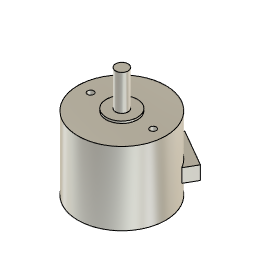
组装01-NIDEC+61mm飞轮 v2 (Autodesk Fusion 360 archive; units mm, degrees)
design "NIDEC无刷电机"
Autodesk Fusion 360 part; units mm, degrees
sketch "草图1" plane through (0, 0, 0) normal (0, 0, 1) x (1, 0, 0)
  circle A0 centre (0, 0) radius 21
  dimension "d1" = 42
  constraint coincident A0.centre origin
  measures "d1" diameter of A0
extrude "拉伸1" add sketch "草图1" along normal blind 35
sketch "草图2" plane through (0, 0, 35) normal (0, 0, 1) x (-1, 0, 0)
  circle A0 centre (0, 0) radius 21
  circle A1 centre (0, 0) radius 3
  dimension "d4" = 6
  constraint coincident A0.centre A1.centre
  measures "d4" diameter of A1
extrude "拉伸2" add sketch "草图2" along normal blind 18 contours A1
sketch "草图3" plane through (0, 0, 35) normal (0, 0, 1) x (-1, 0, 0)
  circle A0 centre (0, 0) radius 3
  circle A1 centre (0, 0) radius 21
  circle A2 centre (0, 0) radius 7.5
  dimension "d7" = 15
  constraint concentric A0 A2
  measures "d7" diameter of A2
extrude "拉伸3" add sketch "草图3" along normal blind 1 contours A2
sketch "草图4" plane through (0, 0, 35) normal (0, 0, 1) x (-1, 0, 0)
  circle A0 centre (0, 0) radius 7.5
  circle A1 centre (0, 0) radius 21
  circle A2 centre (0, 0) radius 15 construction
  circle A3 centre (15, -0.038) radius 1.5
  circle A4 centre (-15, 0) radius 1.5
  dimension "d10" = 30
  dimension "d11" = 3
  dimension "d12" = 3
  constraint coincident A0.centre A1.centre
  constraint coincident A2 A3.centre
  constraint coincident A2 A4.centre
  measures "d10" diameter of A2
  measures "d11" diameter of A3
  measures "d12" diameter of A4
extrude "拉伸4" cut sketch "草图4" against normal blind 10 contours A3 | A4
sketch "草图5" plane through (0, 0, 35) normal (0, 0, 1) x (-1, 0, 0)
  circle A0 centre (-15, 0) radius 1.5
  circle A1 centre (15, -0.038) radius 1.5
  circle A2 centre (0, 0) radius 7.5
  circle A3 centre (0, 0) radius 21
  line L0 (0, 0) -> (-15, 0) construction
  line L1 (-10.4937, -18.1902) -> (0, 0) construction
  line L2 (-0.5625, -20.9925) -> (-3.4002, -26.8403)
  line L3 (-3.4002, -26.8403) -> (-21.1573, -16.5965)
  line L4 (-21.1573, -16.5965) -> (-17.9093, -10.9662)
  dimension "d16" = 60.02
  dimension "d17" = 6.5
  dimension "d18" = 20.5
  constraint coincident A2.centre A3.centre
  constraint coincident A0.centre L0.end
  constraint coincident A3 L1.start
  constraint coincident A3 L2.start
  constraint coincident A3 L4.end
  constraint equal L2 L4
  constraint parallel L1 L4
  constraint perpendicular L1 L3
  measures "d16" angle of L0 L1
  measures "d17" distance of L2.start L2.end
  measures "d18" distance of L2.end L3.end
ref_plane "工作平面2" through (0, 0, 15) normal (0, 0, -1) x (-1, 0, 0)
sketch "草图6" plane through (0, 0, 15) normal (0, 0, -1) x (1, 0, 0)
  line L0 (10.2887, -17.835) -> (0, 0)
  line L1 (0, 0) -> (15, 0)
  line L2 (0.2802, -20.9981) -> (3.5282, -26.6284)
  line L3 (3.5282, -26.6284) -> (21.2853, -16.3846)
  line L4 (18.0373, -10.7543) -> (21.2853, -16.3846)
  circle A0 centre (0, 0) radius 21
  dimension "d23" = 60.02
  dimension "d24" = 6.5
  dimension "d25" = 6.5
  dimension "d26" = 20.5
  constraint coincident L0.end L1.start
  constraint horizontal L1
  constraint parallel L2 L4
  constraint parallel L0 L2
  constraint perpendicular L0 L3
  constraint coincident L2.start A0
  constraint coincident L4.start A0
  measures "d23" angle of L0 L1
  measures "d24" distance of L2.start L2.end
  measures "d25" distance of L3.end L4.start
  measures "d26" distance of L2.end L3.end
extrude "拉伸6" add sketch "草图6" along normal blind 6.5 contours L2 L3 L4 A0

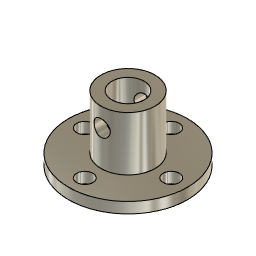
design "联轴器-6mm孔径"
Autodesk Fusion 360 part; units mm, degrees
sketch "草图1" plane through (0, 0, 0) normal (0, 0, 1) x (1, 0, 0)
  circle A0 centre (0, 0) radius 11
  dimension "d1" = 22
  constraint coincident A0.centre origin
  measures "d1" diameter of A0
extrude "拉伸1" add sketch "草图1" along normal blind 2
sketch "草图2" plane through (0, 0, 2) normal (0, 0, 1) x (-1, 0, 0)
  circle A0 centre (0, 0) radius 11
  circle A1 centre (0, 0) radius 5
  constraint concentric A0 A1
extrude "拉伸2" add sketch "草图2" along normal blind 10 contours A1
sketch "草图3" plane through (0, 0, 12) normal (0, 0, 1) x (-1, 0, 0)
  circle A0 centre (0, 0) radius 5
  circle A1 centre (0, 0) radius 3
  dimension "d6" = 6
  constraint concentric A0 A1
  measures "d6" diameter of A1
extrude "拉伸3" cut sketch "草图3" against normal blind 12 contours A1
sketch "草图4" plane through (0, 0, 2) normal (0, 0, 1) x (-1, 0, 0)
  circle A0 centre (0, 0) radius 5
  circle A1 centre (0, 0) radius 11
  circle A2 centre (0, 0) radius 8 construction
  circle A3 centre (8, 0.0048) radius 1.5
  circle A4 centre (-0.0048, 8) radius 1.5
  circle A5 centre (-8, -0.0048) radius 1.5
  circle A6 centre (0.0048, -8) radius 1.5
  dimension "d9" = 16
  dimension "d10" = 3
  dimension "d12" = 360
  constraint coincident A0.centre A1.centre
  constraint coincident A2 A3.centre
  measures "d9" diameter of A2
  measures "d10" diameter of A3
extrude "拉伸4" cut sketch "草图4" against normal blind 2 contours A3 | A4 | A5 | A6
sketch "草图5" plane through (0, 0, 0) normal (0, 1, 0) x (1, 0, 0)
  circle A0 centre (0, -8.5) radius 1.5
  dimension "d15" = 3
  measures "d15" diameter of A0
extrude "拉伸5" cut sketch "草图5" along normal mid plane 11

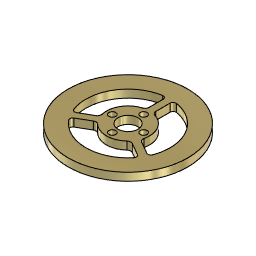
design "惯性飞轮-61mm直径"
Autodesk Fusion 360 part; units mm, degrees
sketch "草图1" plane through (0, 0, 0) normal (0, 0, 1) x (1, 0, 0)
  circle A0 centre (0, 0) radius 30.5
  circle A1 centre (-8, 0) radius 1.75
  line L0 (0, 0) -> (-11, 0)
  circle A2 centre (0, 0) radius 5.1
  circle A3 centre (0, -8) radius 1.75
  circle A4 centre (8, 0) radius 1.75
  circle A5 centre (0, 8) radius 1.75
  line L1 (-1.75, 21.4287) -> (-1.75, 10.8599)
  line L2 (1.75, 21.4287) -> (1.75, 10.8599)
  line L3 (-17.6828, -12.2299) -> (-8.53, -6.9455)
  line L4 (19.4328, -9.1988) -> (10.28, -3.9144)
  line L5 (-19.4328, -9.1988) -> (-10.28, -3.9144)
  line L6 (17.6828, -12.2299) -> (8.53, -6.9455)
  arc A6 (19.4328, -9.1988) -> (1.75, 21.4287) centre (0, 0) ccw
  arc A7 (-1.75, 21.4287) -> (-19.4328, -9.1988) centre (0, 0) ccw
  arc A8 (-17.6828, -12.2299) -> (17.6828, -12.2299) centre (0, 0) ccw
  arc A9 (-8.53, -6.9455) -> (8.53, -6.9455) centre (0, 0) ccw
  arc A10 (10.28, -3.9144) -> (1.75, 10.8599) centre (0, 0) ccw
  arc A11 (-1.75, 10.8599) -> (-10.28, -3.9144) centre (0, 0) ccw
  dimension "d1" = 61
  dimension "d2" = 43
  dimension "d3" = 22
  dimension "d4" = 3.5
  dimension "d5" = 10.2
  dimension "d6" = 8
  dimension "d8" = 360
  dimension "d9" = 3.5
  dimension "d12" = 360
  dimension "d14" = 360
  constraint coincident A0.centre L0.start
  constraint concentric A7 A9
  constraint coincident L0.end A9
  constraint horizontal L0
  constraint coincident A1.centre L0
  constraint concentric A2 A9
  constraint coincident L1.end A9
  constraint vertical L1
  constraint coincident L2.end A9
  constraint parallel L1 L2
  constraint concentric A6 A7
  constraint concentric A7 A8
  constraint concentric A9 A10
  constraint concentric A10 A11
  measures "d1" diameter of A0
  measures "d2" diameter of A7
  measures "d3" diameter of A9
  measures "d4" diameter of A1
  measures "d5" diameter of A2
  measures "d6" distance of A1.centre A0.centre
  measures "d9" distance of L1 L2
extrude "拉伸1" add sketch "草图1" along normal blind 4
fillet "圆角1" radius 2 2 edges at (8.53, -6.9455, 2) (-8.53, -6.9455, 2)
fillet "圆角2" radius 2 4 edges at (10.28, -3.9144, 2) (1.75, 10.8599, 2) (-1.75, 10.8599, 2) (-10.28, -3.9144, 2)
fillet "圆角3" radius 1.5 6 edges at (-1.75, 21.4287, 2) (17.6828, -12.2299, 2) (-19.4328, -9.1988, 2) (19.4328, -9.1988, 2) (-17.6828, -12.2299, 2) (1.75, 21.4287, 2)
